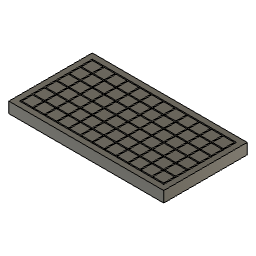
Tile Display v3 (Autodesk Fusion 360 design; units mm, degrees)
Autodesk Fusion 360 part; units mm, degrees
note: some values were not read from the file. Chosen so that the rebuilt part matches the saved one: which bodies a step acts on.
sketch "Sketch1" plane through (0, 0, 0) normal (0, 0, 1) x (1, 0, 0)
  line L0 (-139.965, 81.2061) -> (146.035, 81.2061)
  line L1 (146.035, 81.2061) -> (146.035, -72.7939)
  line L2 (146.035, -72.7939) -> (-139.965, -72.7939)
  line L3 (-139.965, -72.7939) -> (-139.965, 81.2061)
  line L4 (136.035, -62.7939) -> (-129.965, -62.7939)
  line L5 (-129.965, -62.7939) -> (-129.965, 71.2061)
  line L6 (-129.965, 71.2061) -> (136.035, 71.2061)
  line L7 (136.035, 71.2061) -> (136.035, -62.7939)
  line L8 (-127.965, 69.2061) -> (134.035, 69.2061)
  line L9 (134.035, 69.2061) -> (134.035, -60.7939)
  line L10 (134.035, -60.7939) -> (-127.965, -60.7939)
  line L11 (-127.965, -60.7939) -> (-127.965, 69.2061)
  line L12 (-127.965, 69.2061) -> (-107.965, 69.2061)
  line L13 (-107.965, 69.2061) -> (-107.965, 49.2061)
  line L14 (-107.965, 49.2061) -> (-127.965, 49.2061)
  line L15 (-127.965, 49.2061) -> (-127.965, 69.2061)
  line L16 (-105.965, 69.2061) -> (-105.965, 47.2061)
  line L17 (-105.965, 47.2061) -> (-127.965, 47.2061)
  line L18 (-105.965, 69.2061) -> (-105.965, -60.7939)
  line L19 (-127.965, 47.2061) -> (134.035, 47.2061)
  line L20 (-107.965, 69.2061) -> (-107.965, -60.7939)
  line L21 (-127.965, 49.2061) -> (134.035, 49.2061)
  line L22 (-127.965, 47.2061) -> (-107.965, 47.2061)
  line L23 (-107.965, 47.2061) -> (-107.965, 27.2061)
  line L24 (-107.965, 27.2061) -> (-127.965, 27.2061)
  line L25 (-127.965, 27.2061) -> (-127.965, 47.2061)
  line L26 (-127.965, 27.2061) -> (134.035, 27.2061)
  line L27 (-127.965, 25.2061) -> (134.035, 25.2061)
  line L28 (-127.965, 5.2061) -> (134.035, 5.2061)
  line L29 (-127.965, -16.7939) -> (134.035, -16.7939)
  line L30 (-127.965, 3.2061) -> (134.035, 3.2061)
  line L31 (-127.965, -38.7939) -> (134.035, -38.7939)
  line L32 (-127.965, -18.7939) -> (134.035, -18.7939)
  line L33 (-127.965, -40.7939) -> (134.035, -40.7939)
  line L34 (-85.965, 69.2061) -> (-85.965, -60.7939)
  line L35 (-83.965, 69.2061) -> (-83.965, -60.7939)
  line L36 (-63.965, 69.2061) -> (-63.965, -60.7939)
  line L37 (-61.965, 69.2061) -> (-61.965, -60.7939)
  line L38 (-41.965, 69.2061) -> (-41.965, -60.7939)
  line L39 (-39.965, 69.2061) -> (-39.965, -60.7939)
  line L40 (-19.965, 69.2061) -> (-19.965, -60.7939)
  line L41 (-17.965, 69.2061) -> (-17.965, -60.7939)
  line L42 (2.035, 69.2061) -> (2.035, -60.7939)
  line L43 (4.035, 69.2061) -> (4.035, -60.7939)
  line L44 (24.035, 69.2061) -> (24.035, -60.7939)
  line L45 (26.035, 69.2061) -> (26.035, -60.7939)
  line L46 (46.035, 69.2061) -> (46.035, -60.7939)
  line L47 (48.035, 69.2061) -> (48.035, -60.7939)
  line L48 (68.035, 69.2061) -> (68.035, -60.7939)
  line L49 (70.035, 69.2061) -> (70.035, -60.7939)
  line L50 (90.035, 69.2061) -> (90.035, -60.7939)
  line L51 (92.035, 69.2061) -> (92.035, -60.7939)
  line L52 (112.035, 69.2061) -> (112.035, -60.7939)
  line L53 (114.035, 69.2061) -> (114.035, -60.7939)
  dimension "d1" = 286
  dimension "d2" = 154
  dimension "d9" = 10
  dimension "d11" = 20
  dimension "d12" = 20
  dimension "d13" = -2
  dimension "d15" = 2
  dimension "d18" = 24
  constraint horizontal L0
  constraint vertical L1
  constraint horizontal L2
  constraint vertical L3
  constraint horizontal L12
  constraint vertical L13
  constraint horizontal L14
  constraint vertical L15
  constraint coincident L10 L18.end
  constraint perpendicular L10 L18
  constraint coincident L9 L19.end
  constraint perpendicular L9 L19
  constraint coincident L10 L20.end
  constraint perpendicular L10 L20
  constraint coincident L9 L21.end
  constraint perpendicular L9 L21
  constraint horizontal L22
  constraint vertical L23
  constraint horizontal L24
  constraint vertical L25
  constraint coincident L9 L26.end
  constraint perpendicular L9 L26
  measures "d1" distance of L0.start L0.end
  measures "d2" distance of L0.start L2.end
  measures "d11" distance of L8.start L12.end
  measures "d12" distance of L8.start L14.end
extrude "Extrude1" add sketch "Sketch1" along normal blind 20 contours L0 L1 L2 L3 makes body 1
extrude "Extrude2" add sketch "Sketch1" along normal blind 20 separate body contours L8 L11 L12 L13 L14 L15 L20 L21 | L8 L16 L18 L21 L34 | L11 L17 L19 L20 L22 L23 L24 L25 L26 | L8 L21 L35 L36 | L18 L19 L26 L34 | L11 L20 L27 L28 | L8 L21 L37 L38 | L19 L26 L35 L36 | L18 L27 L28 L34 | L11 L20 L29 L30 | L8 L21 L39 L40 | L19 L26 L37 L38 | L27 L28 L35 L36 | L18 L29 L30 L34 | L11 L20 L31 L32 | L8 L21 L41 L42 | L19 L26 L39 L40 | L27 L28 L37 L38 | L29 L30 L35 L36 | L18 L31 L32 L34 | L10 L11 L20 L33 | L8 L21 L43 L44 | L19 L26 L41 L42 | L27 L28 L39 L40 | L29 L30 L37 L38 | L31 L32 L35 L36 | L10 L18 L33 L34 | L8 L21 L45 L46 | L19 L26 L43 L44 | L27 L28 L41 L42 | L29 L30 L39 L40 | L31 L32 L37 L38 | L10 L33 L35 L36 | L8 L21 L47 L48 | L19 L26 L45 L46 | L27 L28 L43 L44 | L29 L30 L41 L42 | L31 L32 L39 L40 | L10 L33 L37 L38 | L8 L21 L49 L50 | L19 L26 L47 L48 | L27 L28 L45 L46 | L29 L30 L43 L44 | L31 L32 L41 L42 | L10 L33 L39 L40 | L8 L21 L51 L52 | L19 L26 L49 L50 | L27 L28 L47 L48 | L29 L30 L45 L46 | L31 L32 L43 L44 | L10 L33 L41 L42 | L8 L9 L21 L53 | L19 L26 L51 L52 | L27 L28 L49 L50 | L29 L30 L47 L48 | L31 L32 L45 L46 | L10 L33 L43 L44 | L9 L19 L26 L53 | L27 L28 L51 L52 | L29 L30 L49 L50 | L31 L32 L47 L48 | L10 L33 L45 L46 | L9 L27 L28 L53 | L29 L30 L51 L52 | L31 L32 L49 L50 | L10 L33 L47 L48 | L9 L29 L30 L53 | L31 L32 L51 L52 | L10 L33 L49 L50 | L9 L31 L32 L53 | L10 L33 L51 L52 | L9 L10 L33 L53 makes body 2 at (98.7016, 18.5395, 0) makes body 3 at (32.7016, 18.5395, 0) makes body 4 at (39.3683, -60.7939, 6.6667) makes body 5 at (76.7016, -18.7939, 6.6667) makes body 6 at (120.7016, -25.4605, 0) makes body 7 at (32.7016, -25.4605, 0) makes body 8 at (-11.2984, 3.2061, 6.6667) makes body 9 at (-19.965, -25.4605, 6.6667) makes body 10 at (-55.2984, 3.2061, 6.6667) makes body 11 at (-77.2984, -18.7939, 6.6667) makes body 12 at (-121.2984, -18.7939, 6.6667) makes body 13 at (-99.2984, 18.5395, 0) makes body 14 at (-77.2984, 47.2061, 6.6667) makes body 15 at (24.035, 62.5395, 6.6667) makes body 16 at (54.7016, 62.5395, 0) makes body 17 at (112.035, 62.5395, 6.6667) makes body 18 at (2.035, 62.5395, 6.6667) makes body 19 at (-85.965, 62.5395, 6.6667) makes body 20 at (-77.2984, 62.5395, 0) makes body 21 at (120.7016, 62.5395, 0) makes body 22 at (90.035, 62.5395, 6.6667) makes body 23 at (46.035, 62.5395, 6.6667) makes body 24 at (-11.2984, 47.2061, 6.6667) makes body 25 at (-105.965, 40.5395, 6.6667) makes body 26 at (-99.2984, 3.2061, 6.6667) makes body 27 at (-121.2984, -40.7939, 6.6667) makes body 28 at (-77.2984, 3.2061, 6.6667) makes body 29 at (-55.2984, -18.7939, 6.6667) makes body 30 at (-19.965, -3.4605, 6.6667) makes body 31 at (-11.2984, -18.7939, 6.6667) makes body 32 at (54.7016, -3.4605, 0) makes body 33 at (98.7016, -40.7939, 6.6667) makes body 34 at (76.7016, -40.7939, 6.6667) makes body 35 at (10.7016, -18.7939, 13.3333) makes body 36 at (10.7016, 18.5395, 0) makes body 37 at (120.7016, 18.5395, 0) makes body 38 at (76.7016, 3.2061, 6.6667) makes body 39 at (32.7016, -3.4605, 0) makes body 40 at (54.7016, -25.4605, 0) makes body 41 at (98.7016, -18.7939, 6.6667) makes body 42 at (98.7016, 3.2061, 6.6667) makes body 43 at (10.7016, -40.7939, 13.3333) makes body 44 at (-11.2984, 18.5395, 0) makes body 45 at (-26.6317, -60.7939, 6.6667) makes body 46 at (-55.2984, 18.5395, 0) makes body 47 at (-77.2984, -40.7939, 6.6667) makes body 48 at (-99.2984, -18.7939, 6.6667) makes body 49 at (-107.965, 18.5395, 13.3333) makes body 50 at (-55.2984, 47.2061, 6.6667) makes body 51 at (10.7016, 47.2061, 13.3333) makes body 52 at (54.7016, 40.5395, 0) makes body 53 at (98.7016, 47.2061, 6.6667) makes body 54 at (-19.965, 62.5395, 6.6667) makes body 55 at (-127.965, 55.8728, 6.6667) makes body 56 at (-41.965, 62.5395, 6.6667) makes body 57 at (120.7016, 40.5395, 0) makes body 58 at (76.7016, 47.2061, 6.6667) makes body 59 at (32.7016, 40.5395, 0) makes body 60 at (-19.965, 40.5395, 6.6667) makes body 61 at (-114.6317, 47.2061, 6.6667) makes body 62 at (-121.2984, 3.2061, 6.6667) makes body 63 at (-99.2984, -40.7939, 6.6667) makes body 64 at (-77.2984, 18.5395, 0) makes body 65 at (-55.2984, -40.7939, 6.6667) makes body 66 at (-19.965, 18.5395, 13.3333) makes body 67 at (-4.6317, -60.7939, 6.6667) makes body 68 at (76.7016, 18.5395, 0) makes body 69 at (127.3683, -60.7939, 6.6667) makes body 70 at (61.3683, -60.7939, 6.6667) makes body 71 at (10.7016, 3.2061, 13.3333) makes body 72 at (61.3683, 11.8728, 0) makes body 73 at (120.7016, -3.4605, 0)
extrude "Extrude3" cut sketch "Sketch1" along normal blind 15 contours L4 L5 L6 L7 | L8 L11 L12 L13 L14 L15 L20 L21 | L8 L13 L16 L18 L20 L21 | L11 L14 L17 L19 L20 L21 L22 | L8 L16 L18 L21 L34 | L16 L17 L18 L19 L20 L21 | L11 L17 L19 L20 L22 L23 L24 L25 L26 | L8 L21 L34 L35 | L16 L18 L19 L21 L34 | L17 L18 L19 L20 L23 L26 | L11 L20 L24 L26 L27 | L8 L21 L35 L36 | L19 L21 L34 L35 | L18 L19 L26 L34 | L18 L20 L26 L27 | L11 L20 L27 L28 | L8 L21 L36 L37 | L19 L21 L35 L36 | L19 L26 L34 L35 | L18 L26 L27 L34 | L18 L20 L27 L28 | L11 L20 L28 L30 | L8 L21 L37 L38 | L19 L21 L36 L37 | L19 L26 L35 L36 | L26 L27 L34 L35 | L18 L27 L28 L34 | L18 L20 L28 L30 | L11 L20 L29 L30 | L8 L21 L38 L39 | L19 L21 L37 L38 | L19 L26 L36 L37 | L26 L27 L35 L36 | L27 L28 L34 L35 | L18 L28 L30 L34 | L18 L20 L29 L30 | L11 L20 L29 L32 | L8 L21 L39 L40 | L19 L21 L38 L39 | L19 L26 L37 L38 | L26 L27 L36 L37 | L27 L28 L35 L36 | L28 L30 L34 L35 | L18 L29 L30 L34 | L18 L20 L29 L32 | L11 L20 L31 L32 | L8 L21 L40 L41 | L19 L21 L39 L40 | L19 L26 L38 L39 | L26 L27 L37 L38 | L27 L28 L36 L37 | L28 L30 L35 L36 | L29 L30 L34 L35 | L18 L29 L32 L34 | L18 L20 L31 L32 | L11 L20 L31 L33 | L8 L21 L41 L42 | L19 L21 L40 L41 | L19 L26 L39 L40 | L26 L27 L38 L39 | L27 L28 L37 L38 | L28 L30 L36 L37 | L29 L30 L35 L36 | L29 L32 L34 L35 | L18 L31 L32 L34 | L18 L20 L31 L33 | L10 L11 L20 L33 | L8 L21 L42 L43 | L19 L21 L41 L42 | L19 L26 L40 L41 | L26 L27 L39 L40 | L27 L28 L38 L39 | L28 L30 L37 L38 | L29 L30 L36 L37 | L29 L32 L35 L36 | L31 L32 L34 L35 | L18 L31 L33 L34 | L10 L18 L20 L33 | L8 L21 L43 L44 | L19 L21 L42 L43 | L19 L26 L41 L42 | L26 L27 L40 L41 | L27 L28 L39 L40 | L28 L30 L38 L39 | L29 L30 L37 L38 | L29 L32 L36 L37 | L31 L32 L35 L36 | L31 L33 L34 L35 | L10 L18 L33 L34 | L8 L21 L44 L45 | L19 L21 L43 L44 | L19 L26 L42 L43 | L26 L27 L41 L42 | L27 L28 L40 L41 | L28 L30 L39 L40 | L29 L30 L38 L39 | L29 L32 L37 L38 | L31 L32 L36 L37 | L31 L33 L35 L36 | L10 L33 L34 L35 | L8 L21 L45 L46 | L19 L21 L44 L45 | L19 L26 L43 L44 | L26 L27 L42 L43 | L27 L28 L41 L42 | L28 L30 L40 L41 | L29 L30 L39 L40 | L29 L32 L38 L39 | L31 L32 L37 L38 | L31 L33 L36 L37 | L10 L33 L35 L36 | L8 L21 L46 L47 | L19 L21 L45 L46 | L19 L26 L44 L45 | L26 L27 L43 L44 | L27 L28 L42 L43 | L28 L30 L41 L42 | L29 L30 L40 L41 | L29 L32 L39 L40 | L31 L32 L38 L39 | L31 L33 L37 L38 | L10 L33 L36 L37 | L8 L21 L47 L48 | L19 L21 L46 L47 | L19 L26 L45 L46 | L26 L27 L44 L45 | L27 L28 L43 L44 | L28 L30 L42 L43 | L29 L30 L41 L42 | L29 L32 L40 L41 | L31 L32 L39 L40 | L31 L33 L38 L39 | L10 L33 L37 L38 | L8 L21 L48 L49 | L19 L21 L47 L48 | L19 L26 L46 L47 | L26 L27 L45 L46 | L27 L28 L44 L45 | L28 L30 L43 L44 | L29 L30 L42 L43 | L29 L32 L41 L42 | L31 L32 L40 L41 | L31 L33 L39 L40 | L10 L33 L38 L39 | L8 L21 L49 L50 | L19 L21 L48 L49 | L19 L26 L47 L48 | L26 L27 L46 L47 | L27 L28 L45 L46 | L28 L30 L44 L45 | L29 L30 L43 L44 | L29 L32 L42 L43 | L31 L32 L41 L42 | L31 L33 L40 L41 | L10 L33 L39 L40 | L8 L21 L50 L51 | L19 L21 L49 L50 | L19 L26 L48 L49 | L26 L27 L47 L48 | L27 L28 L46 L47 | L28 L30 L45 L46 | L29 L30 L44 L45 | L29 L32 L43 L44 | L31 L32 L42 L43 | L31 L33 L41 L42 | L10 L33 L40 L41 | L8 L21 L51 L52 | L19 L21 L50 L51 | L19 L26 L49 L50 | L26 L27 L48 L49 | L27 L28 L47 L48 | L28 L30 L46 L47 | L29 L30 L45 L46 | L29 L32 L44 L45 | L31 L32 L43 L44 | L31 L33 L42 L43 | L10 L33 L41 L42 | L8 L21 L52 L53 | L19 L21 L51 L52 | L19 L26 L50 L51 | L26 L27 L49 L50 | L27 L28 L48 L49 | L28 L30 L47 L48 | L29 L30 L46 L47 | L29 L32 L45 L46 | L31 L32 L44 L45 | L31 L33 L43 L44 | L10 L33 L42 L43 | L8 L9 L21 L53 | L19 L21 L52 L53 | L19 L26 L51 L52 | L26 L27 L50 L51 | L27 L28 L49 L50 | L28 L30 L48 L49 | L29 L30 L47 L48 | L29 L32 L46 L47 | L31 L32 L45 L46 | L31 L33 L44 L45 | L10 L33 L43 L44 | L9 L19 L21 L53 | L19 L26 L52 L53 | L26 L27 L51 L52 | L27 L28 L50 L51 | L28 L30 L49 L50 | L29 L30 L48 L49 | L29 L32 L47 L48 | L31 L32 L46 L47 | L31 L33 L45 L46 | L10 L33 L44 L45 | L9 L19 L26 L53 | L26 L27 L52 L53 | L27 L28 L51 L52 | L28 L30 L50 L51 | L29 L30 L49 L50 | L29 L32 L48 L49 | L31 L32 L47 L48 | L31 L33 L46 L47 | L10 L33 L45 L46 | L9 L26 L27 L53 | L27 L28 L52 L53 | L28 L30 L51 L52 | L29 L30 L50 L51 | L29 L32 L49 L50 | L31 L32 L48 L49 | L31 L33 L47 L48 | L10 L33 L46 L47 | L9 L27 L28 L53 | L28 L30 L52 L53 | L29 L30 L51 L52 | L29 L32 L50 L51 | L31 L32 L49 L50 | L31 L33 L48 L49 | L10 L33 L47 L48 | L9 L28 L30 L53 | L29 L30 L52 L53 | L29 L32 L51 L52 | L31 L32 L50 L51 | L31 L33 L49 L50 | L10 L33 L48 L49 | L9 L29 L30 L53 | L29 L32 L52 L53 | L31 L32 L51 L52 | L31 L33 L50 L51 | L10 L33 L49 L50 | L9 L29 L32 L53 | L31 L32 L52 L53 | L31 L33 L51 L52 | L10 L33 L50 L51 | L9 L31 L32 L53 | L31 L33 L52 L53 | L10 L33 L51 L52 | L9 L31 L33 L53 | L10 L33 L52 L53 | L9 L10 L33 L53 bodies 2 3 4 5 6 7 8 9 10 11 12 13 14 15 16 17 18 19 20 21 22 23 24 25 26 27 28 29 30 31 32 33 34 35 36 37 38 39 40 41 42 43 44 45 46 47 48 49 50 51 52 53 54 55 56 57 58 59 60 61 62 63 64 65 66 67 68 69 70 71 72 73
extrude "Extrude4" add sketch "Sketch1" along normal blind 5 separate body contours L4 L5 L6 L7 | L8 L11 L12 L13 L14 L15 L20 L21 | L8 L13 L16 L18 L20 L21 | L11 L14 L17 L19 L20 L21 L22 | L8 L16 L18 L21 L34 | L16 L17 L18 L19 L20 L21 | L11 L17 L19 L20 L22 L23 L24 L25 L26 | L8 L21 L34 L35 | L16 L18 L19 L21 L34 | L17 L18 L19 L20 L23 L26 | L11 L20 L24 L26 L27 | L8 L21 L35 L36 | L19 L21 L34 L35 | L18 L19 L26 L34 | L18 L20 L26 L27 | L11 L20 L27 L28 | L8 L21 L36 L37 | L19 L21 L35 L36 | L19 L26 L34 L35 | L18 L26 L27 L34 | L18 L20 L27 L28 | L11 L20 L28 L30 | L8 L21 L37 L38 | L19 L21 L36 L37 | L19 L26 L35 L36 | L26 L27 L34 L35 | L18 L27 L28 L34 | L18 L20 L28 L30 | L11 L20 L29 L30 | L8 L21 L38 L39 | L19 L21 L37 L38 | L19 L26 L36 L37 | L26 L27 L35 L36 | L27 L28 L34 L35 | L18 L28 L30 L34 | L18 L20 L29 L30 | L11 L20 L29 L32 | L8 L21 L39 L40 | L19 L21 L38 L39 | L19 L26 L37 L38 | L26 L27 L36 L37 | L27 L28 L35 L36 | L28 L30 L34 L35 | L18 L29 L30 L34 | L18 L20 L29 L32 | L11 L20 L31 L32 | L8 L21 L40 L41 | L19 L21 L39 L40 | L19 L26 L38 L39 | L26 L27 L37 L38 | L27 L28 L36 L37 | L28 L30 L35 L36 | L29 L30 L34 L35 | L18 L29 L32 L34 | L18 L20 L31 L32 | L11 L20 L31 L33 | L8 L21 L41 L42 | L19 L21 L40 L41 | L19 L26 L39 L40 | L26 L27 L38 L39 | L27 L28 L37 L38 | L28 L30 L36 L37 | L29 L30 L35 L36 | L29 L32 L34 L35 | L18 L31 L32 L34 | L18 L20 L31 L33 | L10 L11 L20 L33 | L8 L21 L42 L43 | L19 L21 L41 L42 | L19 L26 L40 L41 | L26 L27 L39 L40 | L27 L28 L38 L39 | L28 L30 L37 L38 | L29 L30 L36 L37 | L29 L32 L35 L36 | L31 L32 L34 L35 | L18 L31 L33 L34 | L10 L18 L20 L33 | L8 L21 L43 L44 | L19 L21 L42 L43 | L19 L26 L41 L42 | L26 L27 L40 L41 | L27 L28 L39 L40 | L28 L30 L38 L39 | L29 L30 L37 L38 | L29 L32 L36 L37 | L31 L32 L35 L36 | L31 L33 L34 L35 | L10 L18 L33 L34 | L8 L21 L44 L45 | L19 L21 L43 L44 | L19 L26 L42 L43 | L26 L27 L41 L42 | L27 L28 L40 L41 | L28 L30 L39 L40 | L29 L30 L38 L39 | L29 L32 L37 L38 | L31 L32 L36 L37 | L31 L33 L35 L36 | L10 L33 L34 L35 | L8 L21 L45 L46 | L19 L21 L44 L45 | L19 L26 L43 L44 | L26 L27 L42 L43 | L27 L28 L41 L42 | L28 L30 L40 L41 | L29 L30 L39 L40 | L29 L32 L38 L39 | L31 L32 L37 L38 | L31 L33 L36 L37 | L10 L33 L35 L36 | L8 L21 L46 L47 | L19 L21 L45 L46 | L19 L26 L44 L45 | L26 L27 L43 L44 | L27 L28 L42 L43 | L28 L30 L41 L42 | L29 L30 L40 L41 | L29 L32 L39 L40 | L31 L32 L38 L39 | L31 L33 L37 L38 | L10 L33 L36 L37 | L8 L21 L47 L48 | L19 L21 L46 L47 | L19 L26 L45 L46 | L26 L27 L44 L45 | L27 L28 L43 L44 | L28 L30 L42 L43 | L29 L30 L41 L42 | L29 L32 L40 L41 | L31 L32 L39 L40 | L31 L33 L38 L39 | L10 L33 L37 L38 | L8 L21 L48 L49 | L19 L21 L47 L48 | L19 L26 L46 L47 | L26 L27 L45 L46 | L27 L28 L44 L45 | L28 L30 L43 L44 | L29 L30 L42 L43 | L29 L32 L41 L42 | L31 L32 L40 L41 | L31 L33 L39 L40 | L10 L33 L38 L39 | L8 L21 L49 L50 | L19 L21 L48 L49 | L19 L26 L47 L48 | L26 L27 L46 L47 | L27 L28 L45 L46 | L28 L30 L44 L45 | L29 L30 L43 L44 | L29 L32 L42 L43 | L31 L32 L41 L42 | L31 L33 L40 L41 | L10 L33 L39 L40 | L8 L21 L50 L51 | L19 L21 L49 L50 | L19 L26 L48 L49 | L26 L27 L47 L48 | L27 L28 L46 L47 | L28 L30 L45 L46 | L29 L30 L44 L45 | L29 L32 L43 L44 | L31 L32 L42 L43 | L31 L33 L41 L42 | L10 L33 L40 L41 | L8 L21 L51 L52 | L19 L21 L50 L51 | L19 L26 L49 L50 | L26 L27 L48 L49 | L27 L28 L47 L48 | L28 L30 L46 L47 | L29 L30 L45 L46 | L29 L32 L44 L45 | L31 L32 L43 L44 | L31 L33 L42 L43 | L10 L33 L41 L42 | L8 L21 L52 L53 | L19 L21 L51 L52 | L19 L26 L50 L51 | L26 L27 L49 L50 | L27 L28 L48 L49 | L28 L30 L47 L48 | L29 L30 L46 L47 | L29 L32 L45 L46 | L31 L32 L44 L45 | L31 L33 L43 L44 | L10 L33 L42 L43 | L8 L9 L21 L53 | L19 L21 L52 L53 | L19 L26 L51 L52 | L26 L27 L50 L51 | L27 L28 L49 L50 | L28 L30 L48 L49 | L29 L30 L47 L48 | L29 L32 L46 L47 | L31 L32 L45 L46 | L31 L33 L44 L45 | L10 L33 L43 L44 | L9 L19 L21 L53 | L19 L26 L52 L53 | L26 L27 L51 L52 | L27 L28 L50 L51 | L28 L30 L49 L50 | L29 L30 L48 L49 | L29 L32 L47 L48 | L31 L32 L46 L47 | L31 L33 L45 L46 | L10 L33 L44 L45 | L9 L19 L26 L53 | L26 L27 L52 L53 | L27 L28 L51 L52 | L28 L30 L50 L51 | L29 L30 L49 L50 | L29 L32 L48 L49 | L31 L32 L47 L48 | L31 L33 L46 L47 | L10 L33 L45 L46 | L9 L26 L27 L53 | L27 L28 L52 L53 | L28 L30 L51 L52 | L29 L30 L50 L51 | L29 L32 L49 L50 | L31 L32 L48 L49 | L31 L33 L47 L48 | L10 L33 L46 L47 | L9 L27 L28 L53 | L28 L30 L52 L53 | L29 L30 L51 L52 | L29 L32 L50 L51 | L31 L32 L49 L50 | L31 L33 L48 L49 | L10 L33 L47 L48 | L9 L28 L30 L53 | L29 L30 L52 L53 | L29 L32 L51 L52 | L31 L32 L50 L51 | L31 L33 L49 L50 | L10 L33 L48 L49 | L9 L29 L30 L53 | L29 L32 L52 L53 | L31 L32 L51 L52 | L31 L33 L50 L51 | L10 L33 L49 L50 | L9 L29 L32 L53 | L31 L32 L52 L53 | L31 L33 L51 L52 | L10 L33 L50 L51 | L9 L31 L32 L53 | L31 L33 L52 L53 | L10 L33 L51 L52 | L9 L31 L33 L53 | L10 L33 L52 L53 | L9 L10 L33 L53 makes body 74
